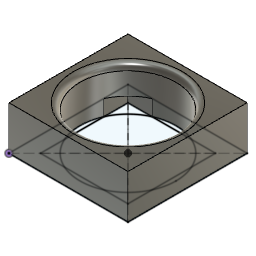
Top Shell - Right Full - Chamfer v2 (Autodesk Fusion 360 archive; units mm, degrees)
design "Encoder Blocker - 7mm"
Autodesk Fusion 360 part; units mm, degrees
sketch "Sketch1" plane through (0, 0, 0) normal (0, 0, 1) x (1, 0, 0)
  line L0 (0, 0) -> (19.05, 0)
  line L1 (19.05, 0) -> (19.05, 19.05)
  line L2 (19.05, 19.05) -> (0, 19.05)
  line L3 (0, 19.05) -> (0, 0)
  line L4 (0, 0) -> (19.05, 19.05) construction
  line L5 (0, 19.05) -> (19.05, 0) construction
  circle A0 centre (9.525, 9.525) radius 7.675
  line L6 (16.525, 2.525) -> (2.525, 2.525)
  line L7 (2.525, 2.525) -> (2.525, 16.525)
  line L8 (2.525, 16.525) -> (16.525, 16.525)
  line L9 (16.525, 16.525) -> (16.525, 2.525)
  line L10 (16.525, 2.525) -> (2.525, 16.525) construction
  line L11 (2.525, 2.525) -> (16.525, 16.525) construction
  point P0 (9.525, 9.525)
  dimension "d1" = 19.05
  dimension "d2" = 19.05
  dimension "d5" = 15.35
  dimension "d6" = 14
  dimension "d7" = 14
  constraint horizontal L0
  constraint vertical L1
  constraint horizontal L2
  constraint vertical L3
  constraint coincident L0.start L3.end
  constraint midpoint L4 P0
  constraint horizontal L6
  constraint perpendicular L6 L7
  constraint parallel L6 L8
  constraint parallel L7 L9
  constraint coincident L10 P0
  constraint coincident L11 P0
  constraint coincident P0 A0.centre
  measures "d1" distance of L0.start L0.end
  measures "d2" distance of L0.start L2.end
  measures "d5" diameter of A0
  measures "d6" distance of L7.end L8.end
  measures "d7" distance of L6.end L7.end
extrude "Extrude1" add sketch "Sketch1" along normal blind 7 contours L0 L1 L2 L3 | A0 L8 L9 | A0 L6 L9 | A0 L7 L8 | A0 L6 L7
extrude "Extrude2" cut sketch "Sketch1" along normal blind 2.5 contours A0 L8 L9 | A0 L6 L9 | A0 L7 L8 | A0 L6 L7
fillet "Fillet1" radius 1 1 edges at (2.3694, 12.3004, 7)
equation "d1 = width"
equation "d2 = height"
equation "encoder_diameter = 15.35 mm"
equation "encoder_cutout = 14 mm"
equation "d5 = encoder_diameter"
equation "d6 = encoder_cutout"
equation "d7 = encoder_cutout"
equation "shell_thickness = 7 mm"
equation "encoder_cut_height = 2.5 mm"
equation "d10 = shell_thickness"
equation "d12 = encoder_cut_height"
equation "height = 19.05 mm"
equation "width = 19.05 mm"
